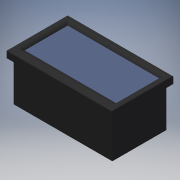
# Autodesk Inventor part: ВольтметрЦифровой
Saved by Autodesk Inventor 2019 (Build 230136000, 136)
## iProperties
Created: 2020-10-19
Part Number: ВольтметрЦифровой
Material: Типовые
Document SubType Name: Modeling
Designer: Surflay
Density: 1 g/cm^3
Appearance: По умолчанию
Author: Surflay
Autodesk Inventor part; units mm, degrees
ref_plane "YZ Plane" through (0, 0, 0) normal (1, 0, 0) x (0, 1, 0)
ref_plane "XZ Plane" through (0, 0, 0) normal (0, 1, 0) x (-1, 0, 0)
ref_plane "XY Plane" through (0, 0, 0) normal (0, 0, 1) x (1, 0, 0)
sketch "Эскиз1" plane through (0, 0, 0) normal (0, 1, 0) x (-1, 0, 0)
  line L0 (0, 0) -> (-45, 0)
  line L1 (-45, 0) -> (-45, -26)
  line L2 (-45, -26) -> (0, -26)
  line L3 (0, -26) -> (0, 0)
  dimension "d0" = 45
  dimension "d1" = 26
  constraints: 8 end point, 2 parallel, 1 horizontal, 1 perpendicular
  measures "d0" distance of L2.end L1.end
  measures "d1" distance of L1.end L0.end
extrude "Выдавливание1" add sketch "Эскиз1" along normal blind 20
sketch "Эскиз2" plane through (0, 20, 0) normal (0, 1, 0) x (1, 0, 0)
  line L0 (3, 3) -> (42, 3)
  line L1 (42, 3) -> (42, 23)
  line L2 (42, 23) -> (3, 23)
  line L3 (3, 23) -> (3, 3)
  line L4 (0, 0) -> (45, 0) projected
  line L5 (0, 26) -> (0, 0) projected
  line L6 (45, 26) -> (0, 26) projected
  line L7 (45, 0) -> (45, 26) projected
  dimension "d4" = 3
  dimension "d5" = 3
  dimension "d6" = 3
  dimension "d7" = 3
  constraints: 8 end point, 2 parallel, 1 horizontal, 1 perpendicular
  measures "d4" distance between parallel lines of L0 L4
  measures "d5" distance between parallel lines of L3 L5
  measures "d6" distance between parallel lines of L2 L6
  measures "d7" distance between parallel lines of L7 L1
extrude "Выдавливание2" cut sketch "Эскиз2" against normal blind 1 contours L3 L2 L1 L0
fillet "Сопряжение1" radius 2 4 edges at (22.5, 20, -23) (3, 20, -13) (22.5, 19, -3) (42, 20, -13)
fillet "Сопряжение1" radius 0.5 4 edges at (45, 20, -13) (22.5, 20, -26) (0, 20, -13) (22.5, 20, 0)
sketch "Эскиз3" plane through (0, 0, 0) normal (0, -1, 0) x (1, 0, 0)
  line L0 (3, -3) -> (42, -3)
  line L1 (42, -3) -> (42, -23)
  line L2 (42, -23) -> (3, -23)
  line L3 (3, -23) -> (3, -3)
  line L4 (0, 0) -> (45, 0) projected
  line L5 (45, -26) -> (0, -26) projected
  line L6 (45, 0) -> (45, -26) projected
  line L7 (0, -26) -> (0, 0) projected
  dimension "d12" = 3
  dimension "d13" = 3
  dimension "d14" = 3
  dimension "d15" = 3
  constraints: 8 end point, 2 parallel, 1 horizontal, 1 perpendicular
  measures "d12" distance between parallel lines of L4 L0
  measures "d13" distance between parallel lines of L5 L2
  measures "d14" distance between parallel lines of L6 L1
  measures "d15" distance between parallel lines of L7 L3
extrude "Выдавливание3" cut sketch "Эскиз3" against normal blind 4 contours L0 L1 L2 L3
sketch "Эскиз4" plane through (0, 0, 0) normal (0, -1, 0) x (1, 0, 0)
  line L0 (3, -3) -> (42, -3) projected
  line L1 (42, -3) -> (42, -23) projected
  line L2 (3, -3) -> (42, -3)
  line L3 (42, -3) -> (42, -23)
  line L4 (42, -23) -> (3, -23)
  line L5 (3, -23) -> (3, -3)
  line L6 (-2.0024, 1.6795) -> (47.8648, 1.6795)
  line L7 (47.8648, 1.6795) -> (47.8648, -29.3906)
  line L8 (47.8648, -29.3906) -> (-2.0024, -29.3906)
  line L9 (-2.0024, -29.3906) -> (-2.0024, 1.6795)
  line L10 (1.5, -24.5) -> (43.5, -24.5)
  line L11 (43.5, -24.5) -> (43.5, -1.5)
  line L12 (43.5, -1.5) -> (1.5, -1.5)
  line L13 (1.5, -1.5) -> (1.5, -24.5)
  point P0 (0, 0)
  dimension "d18" = 1.5
  dimension "d19" = 1.5
  dimension "d20" = 1.5
  dimension "d21" = 1.5
  constraints: 24 end point, 6 parallel, 3 horizontal, 3 perpendicular
  measures "d18" distance between parallel lines of L12 L0
  measures "d19" distance between parallel lines of L13 L5
  measures "d20" distance between parallel lines of L4 L10
  measures "d21" distance between parallel lines of L11 L1
extrude "Выдавливание4" cut sketch "Эскиз4" against normal blind 17 contours L6 L7 L8 L9
